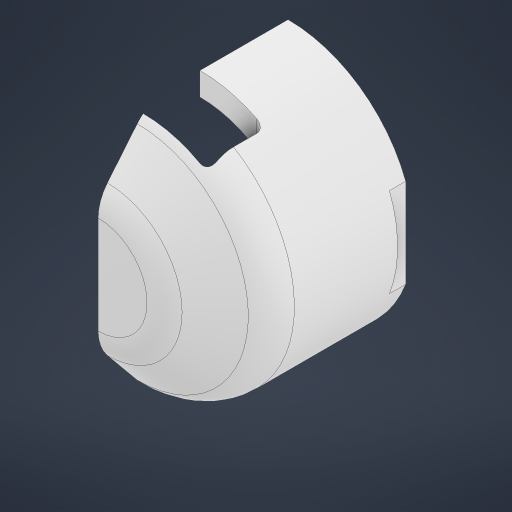
# Autodesk Inventor part: EncCoverHalf
Saved by Autodesk Inventor 2023 (Build 270158000, 158)
## iProperties
Created: 2023-10-08
Part Number: EncCoverHalf
Material: Пластик ПАЭК
Document SubType Name: Modeling
Designer: khrip
Density: 1.32 g/cm^3
Appearance: Гладкий — белый
Author: khrip
Autodesk Inventor part; units mm, degrees
ref_plane "YZ Plane" through (0, 0, 0) normal (1, 0, 0) x (0, 1, 0)
ref_plane "XZ Plane" through (0, 0, 0) normal (0, 1, 0) x (-1, 0, 0)
sketch "Эскиз1" plane through (0, 0, 0) normal (1, 0, 0) x (0, 1, 0)
  line L0 (0, 1) -> (-7.8216, 1)
  line L1 (-7.8216, 1) -> (-7.8216, 3.85)
  line L2 (-7.8216, 3.85) -> (0, 3.85)
  line L3 (0, 3.85) -> (0, 1)
  line L4 (-15.5, -46.55) -> (-15.5, -19.55)
  line L5 (-15.5, -19.55) -> (-12.65, -19.55)
  line L6 (-12.65, -19.55) -> (-12.65, -2.466)
  line L7 (-12.65, -2.466) -> (-15.5, -2.466)
  line L8 (-15.5, -2.466) -> (-15.5, -19.55)
  line L9 (-12.15, -9.434) -> (-12.15, -39.916)
  line L10 (-15.5, -2.466) -> (-7.8216, 3.85)
  line L11 (-7.8216, 3.85) -> (-6.0111, 1.649)
  line L12 (-6.0111, 1.649) -> (-13.6895, -4.6671)
  line L13 (-13.6895, -4.6671) -> (-15.5, -2.466)
  line L14 (-6.8, -2) -> (-6.8, -7.7)
  line L15 (0, -56.63) -> (0, 13.93) projected
  point P0 (0, 0)
  point P1 (-6.8, 1)
  point P2 (-12.65, -3.812)
  dimension "d0" = 0.5
  dimension "d1" = 2.85
  dimension "d2" = 2.85
  dimension "d3" = 50.56
  dimension "d4" = 0
  dimension "d5" = 1
  dimension "d6" = 2.85
  dimension "d7" = 0
  constraints: 30 end point, 6 parallel, 3 perpendicular, 3 vertical, 2 horizontal, 2 point on line, 6 other
  measures "d0" distance between parallel lines of L6 L9
  measures "d1" distance between parallel lines of L8 L6
  measures "d2" distance between parallel lines of L12 L10
  measures "d3" angle of L8 L10
  measures "d4" distance from line of point (0, 0) L3
  measures "d5" distance from line of L0 point (0, 0)
  measures "d6" distance between parallel lines of L2 L0
  measures "d7" distance from line of L14 point (-6.8, 1)
revolve "Вращение1" add sketch "Эскиз1" angle 180 about axis through (0, 0, -10) along (0, 0, 1)
ref_plane "РабПлоскость1" through (7, 16.35, -7.7) normal (0, 1, 0) x (-1, 0, 0)
sketch "Эскиз2" plane through (7, 16.35, -7.7) normal (0, 1, 0) x (-1, 0, 0)
  line L0 (0, 0) -> (14, 0) projected
  line L1 (14, 0) -> (14, 5) projected
  line L2 (0, 5) -> (14, 5) projected
  line L3 (0, 0) -> (0, 5) projected
  line L4 (0, -1) -> (14, -1)
  line L5 (15, 0) -> (15, 5)
  line L6 (14, 6) -> (0, 6)
  line L7 (-1, 5) -> (-1, 0)
  arc A0 (-1, 0) -> (0, -1) centre (0, 0) ccw
  arc A1 (0, 6) -> (-1, 5) centre (0, 5) ccw
  arc A2 (15, 5) -> (14, 6) centre (14, 5) ccw
  arc A3 (14, -1) -> (15, 0) centre (14, 0) ccw
  point P0 (7, 7.7)
  dimension "d9" = 1
  dimension "d10" = 1
  dimension "d11" = 1
  dimension "d12" = 1
  dimension "d13" = 1
  dimension "d14" = 1
  constraints: 8 end point, 8 point on circle, 8 tangent, 4 centre point, 2 equal radius, 2 parallel, 1 horizontal, 1 perpendicular
  measures "d9" distance between parallel lines of L6 L2
  measures "d10" distance between parallel lines of L0 L4
  measures "d11" distance between parallel lines of L7 L3
  measures "d12" distance between parallel lines of L1 L5
  measures "d13" radius of A0
  measures "d14" radius of A1
extrude "Выдавливание1" cut sketch "Эскиз2" against normal blind 10 contours L3 L2 L1 L0 | A0 L7 A1 L6 A2 L5 A3 L4
fillet "Сопряжение1" radius 5 4 edges at (7.8216, 0, 3.85) (14.938, -4.1361, -2.466) (6.8, 0, 1) (11.916, -4.2464, -3.812)
sketch "Эскиз3" plane through (0, -15.5, -19.55) normal (0, 0, -1) x (-1, 0, 0)
  line L0 (-14.4918, 10.0011) -> (-14.4918, 20.9989) projected
  arc A0 (-14.4918, 20.9989) -> (-14.4918, 10.0011) centre (0, 15.5) ccw projected
  point P0 (0, 15.5)
extrude "Выдавливание2" cut sketch "Эскиз3" against normal blind 2
